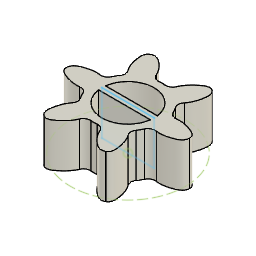
Mini-gear (Autodesk Fusion 360 design; units mm, degrees)
description: Spur Gear; Module: 2.2; Num Teeth: 6; Pressure Angle: 25.0; Backlash: 0.80 mm
Autodesk Fusion 360 part; units mm, degrees
sketch "Esboço4" plane through (0, 0, 0) normal (0, 1, 0) x (1, 0, 0)
  line L0 (-3, -5) -> (3, -5)
  line L1 (3, -5) -> (3, 0)
  line L2 (3, 0) -> (-3, 0)
  line L3 (-3, 0) -> (-3, -5)
  constraint horizontal L0
  constraint perpendicular L0 L1
  constraint perpendicular L1 L2
  constraint perpendicular L0 L3
sketch "Esboço6" plane through (0, 0, 0) normal (0, 1, 0) x (1, 0, 0)
  line L0 (-3, -5) -> (3, -5)
  line L1 (3, -5) -> (3, 0)
  line L2 (3, 0) -> (-3, 0)
  line L3 (-3, 0) -> (-3, -5)
  constraint horizontal L0
  constraint vertical L1
  constraint horizontal L2
  constraint vertical L3
sketch "Esboço1" plane through (0, 0, 0) normal (0, 0, 1) x (1, 0, 0) in component "Spur Gear (6 teeth) (1)"
  circle A0 centre (0, 0) radius 3.9092
  circle A1 centre (0, 0) radius 3
extrude "Extrusão1" add sketch "Esboço1" along normal blind 5 in component "Spur Gear (6 teeth) (1)"
sketch "Esboço2" plane through (0, 0, 0) normal (0, 0, 1) x (1, 0, 0) in component "Spur Gear (6 teeth) (1)"
  spline S0 degree 5 poles (4.1943, -1.1244) (4.2025, -1.1266) (4.219, -1.1311) (4.2435, -1.1382) (4.2762, -1.1481) (4.3172, -1.1607) (4.3585, -1.1727) (4.4003, -1.1831) (4.4429, -1.1916) (4.4862, -1.1981) (4.53, -1.2029) (4.5743, -1.2065) (4.6188, -1.2093) (4.6634, -1.2117) (4.7082, -1.2135) (4.7531, -1.2149) (4.7982, -1.2156) (4.8435, -1.2155) (4.889, -1.2145) (4.9348, -1.2126) (4.9808, -1.2098) (5.0269, -1.2063) (5.0732, -1.2022) (5.1196, -1.1974) (5.1661, -1.1921) (5.2127, -1.1861) (5.2594, -1.1796) (5.3061, -1.1724) (5.353, -1.1645) (5.4, -1.156) (5.4471, -1.1468) (5.4942, -1.1368) (5.5414, -1.1263) (5.5887, -1.1151) (5.636, -1.1034) (5.6833, -1.0912) (5.7307, -1.0786) (5.778, -1.0654) (5.8253, -1.0517) (5.8727, -1.0373) (5.9201, -1.0221) (5.9677, -1.0061) (6.0153, -0.9892) (6.0629, -0.9716) (6.1105, -0.9537) (6.1578, -0.9357) (6.205, -0.9179) (6.252, -0.9003) (6.2989, -0.8824) (6.3458, -0.8637) (6.393, -0.8433) (6.4406, -0.8206) (6.4886, -0.7952) (6.5367, -0.7671) (6.5845, -0.7371) (6.6314, -0.7058) (6.6768, -0.6742) (6.7202, -0.6428) (6.7611, -0.6116) (6.7993, -0.5796) (6.8349, -0.5457) (6.8679, -0.5085) (6.8984, -0.4668) (6.9266, -0.4204) (6.9523, -0.3699) (6.9756, -0.3168) (6.9961, -0.263) (7.0137, -0.2106) (7.0282, -0.1615) (7.0395, -0.1171) (7.0475, -0.0783) (7.0512, -0.0521) (7.0525, -0.0351) (7.0528, -0.025) (7.0527, -0.0203) knots 0 0 0 0 0 0 0.01428571 0.02857143 0.04285714 0.05714286 0.07142857 0.08571429 0.1 0.11428571 0.12857143 0.14285714 0.15714286 0.17142857 0.18571429 0.2 0.21428571 0.22857143 0.24285714 0.25714286 0.27142857 0.28571429 0.3 0.31428571 0.32857143 0.34285714 0.35714286 0.37142857 0.38571429 0.4 0.41428571 0.42857143 0.44285714 0.45714286 0.47142857 0.48571429 0.5 0.51428571 0.52857143 0.54285714 0.55714286 0.57142857 0.58571429 0.6 0.61428571 0.62857143 0.64285714 0.65714286 0.67142857 0.68571429 0.7 0.71428571 0.72857143 0.74285714 0.75714286 0.77142857 0.78571429 0.8 0.81428571 0.82857143 0.84285714 0.85714286 0.87142857 0.88571429 0.9 0.91428571 0.92857143 0.94285714 0.95714286 0.97142857 0.98571429 1 1 1 1 1 1
  spline S1 degree 5 poles (4.098, 1.0988) (4.1063, 1.101) (4.1228, 1.1055) (4.1475, 1.1128) (4.1803, 1.1233) (4.2212, 1.1368) (4.2625, 1.1496) (4.3045, 1.161) (4.3472, 1.1702) (4.3907, 1.1773) (4.4348, 1.1827) (4.4793, 1.1868) (4.5241, 1.1902) (4.569, 1.1931) (4.6141, 1.1957) (4.6592, 1.1977) (4.7046, 1.1991) (4.7502, 1.1996) (4.7961, 1.1991) (4.8422, 1.1978) (4.8886, 1.1956) (4.9351, 1.1927) (4.9817, 1.1892) (5.0285, 1.185) (5.0754, 1.1803) (5.1224, 1.1749) (5.1695, 1.1689) (5.2167, 1.1622) (5.264, 1.1548) (5.3114, 1.1467) (5.359, 1.1381) (5.4066, 1.1288) (5.4543, 1.1189) (5.502, 1.1084) (5.5498, 1.0973) (5.5976, 1.0856) (5.6454, 1.0732) (5.6933, 1.0602) (5.7411, 1.0466) (5.7891, 1.0325) (5.8371, 1.0178) (5.8852, 1.0027) (5.9333, 0.9871) (5.9815, 0.9709) (6.0295, 0.954) (6.0775, 0.9364) (6.1252, 0.918) (6.1728, 0.8989) (6.2203, 0.8792) (6.2679, 0.8591) (6.3158, 0.8389) (6.3641, 0.8187) (6.4127, 0.7984) (6.4614, 0.7778) (6.5098, 0.7563) (6.5575, 0.7335) (6.604, 0.7086) (6.649, 0.6813) (6.6925, 0.6514) (6.7345, 0.619) (6.7751, 0.5842) (6.8146, 0.5475) (6.8529, 0.5091) (6.8897, 0.4692) (6.9245, 0.4279) (6.9566, 0.3852) (6.9852, 0.341) (7.0096, 0.2952) (7.029, 0.2477) (7.0431, 0.1984) (7.0516, 0.1472) (7.0539, 0.1048) (7.0531, 0.0722) (7.0513, 0.0501) (7.0502, 0.039) knots 0 0 0 0 0 0 0.01428571 0.02857143 0.04285714 0.05714286 0.07142857 0.08571429 0.1 0.11428571 0.12857143 0.14285714 0.15714286 0.17142857 0.18571429 0.2 0.21428571 0.22857143 0.24285714 0.25714286 0.27142857 0.28571429 0.3 0.31428571 0.32857143 0.34285714 0.35714286 0.37142857 0.38571429 0.4 0.41428571 0.42857143 0.44285714 0.45714286 0.47142857 0.48571429 0.5 0.51428571 0.52857143 0.54285714 0.55714286 0.57142857 0.58571429 0.6 0.61428571 0.62857143 0.64285714 0.65714286 0.67142857 0.68571429 0.7 0.71428571 0.72857143 0.74285714 0.75714286 0.77142857 0.78571429 0.8 0.81428571 0.82857143 0.84285714 0.85714286 0.87142857 0.88571429 0.9 0.91428571 0.92857143 0.94285714 0.95714286 0.97142857 0.98571429 1 1 1 1 1 1
  arc A0 (7.0527, -0.0203) -> (7.0502, 0.039) centre (-9.0164, -0.669) ccw
  line L0 (3.7667, -1.0105) -> (4.1943, -1.1244)
  line L1 (3.7667, 1.0105) -> (4.098, 1.0988)
  line L2 (3.7667, -1.0105) -> (3.7667, 1.0105)
  point P0 (4.3908, -1.1804)
  point P1 (4.6003, -1.2081)
  point P2 (4.8184, -1.2154)
  point P3 (5.0431, -1.2048)
  point P4 (5.2732, -1.1774)
  point P5 (5.5078, -1.1337)
  point P6 (5.7458, -1.0743)
  point P7 (5.9864, -0.9993)
  point P8 (6.229, -0.9089)
  point P9 (6.4727, -0.8032)
  point P10 (6.7195, -0.6429)
  point P11 (6.9009, -0.4611)
  point P12 (7.0198, -0.189)
  point P13 (4.2936, 1.1577)
  point P14 (4.5027, 1.1885)
  point P15 (4.7207, 1.1991)
  point P16 (4.9455, 1.1918)
  point P17 (5.176, 1.1678)
  point P18 (5.4112, 1.1277)
  point P19 (5.65, 1.0718)
  point P20 (5.8918, 1.0004)
  point P21 (6.1357, 0.9137)
  point P22 (6.381, 0.8116)
  point P23 (6.6268, 0.6944)
  point P24 (6.8411, 0.5204)
  point P25 (7.0056, 0.3005)
extrude "Extrusão2" add sketch "Esboço2" along normal blind 5 in component "Spur Gear (6 teeth) (1)"
fillet "Arredondamento1" radius 0.8 2 edges at (3.7757, -1.0129, 2.5) (3.7757, 1.0129, 2.5) in component "Spur Gear (6 teeth) (1)"
pattern_circular "Padrão circular1" count 6 over 360 about axis through (0, 0, 0) along (0, 0, 1) of "Extrusão2", "Arredondamento1" in component "Spur Gear (6 teeth) (1)"
sketch "Esboço3" plane through (0, 0, 0) normal (0, 0, 1) x (1, 0, 0) in component "Spur Gear (6 teeth) (1)"
  circle A0 centre (0, 0) radius 6.6 construction
extrude "Extrusão3" add sketch "Esboço6" along normal mid plane 0.8 in component "Spur Gear (6 teeth) (1)"
sketch "Esboço3 (2)" plane through (0, 0, 0) normal (1, 0, 0) x (0, 1, 0)
  line L0 (-3, 5) -> (3, 5)
  line L1 (3, 5) -> (3, 0)
  line L2 (3, 0) -> (-3, 0)
  line L3 (-3, 0) -> (-3, 5)
  constraint horizontal L0
  constraint perpendicular L0 L1
  constraint perpendicular L1 L2
  constraint perpendicular L0 L3
component "Spur Gear (6 teeth) (1)" placed x (1, 0, 0) y (0, 1, 0) z (0, 0, 1) at (0, 0, 0)
